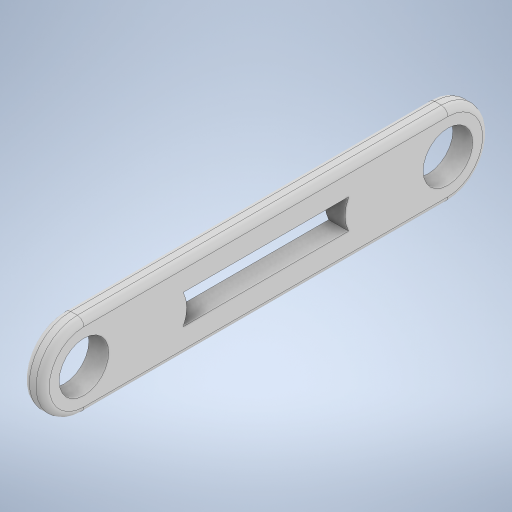
# Autodesk Inventor part: FemurHornSide
Saved by Autodesk Inventor 2024 (Build 280153000, 153)
## iProperties
Created: 2026-01-07
Part Number: FemurHornSide
Material: Generic
Document SubType Name: Modeling
Designer: Liam
Density: 1 g/cm^3
Appearance: Default
Mass: 26.103 g
Surface Area: 91.6684 cm^2
Volume: 26.103 cm^3
Author: Liam
Autodesk Inventor part; units mm, degrees
ref_plane "YZ Plane" through (0, 0, 0) normal (1, 0, 0) x (0, 1, 0)
ref_plane "XZ Plane" through (0, 0, 0) normal (0, 1, 0) x (-1, 0, 0)
ref_plane "XY Plane" through (0, 0, 0) normal (0, 0, 1) x (1, 0, 0)
sketch "Sketch1" plane through (0, 0, 0) normal (1, 0, 0) x (0, 1, 0)
  line L0 (12.5, 55) -> (-12.5, 55)
  line L1 (-12.5, 55) -> (-12.5, -55)
  line L2 (-12.5, -55) -> (12.5, -55)
  line L3 (12.5, -55) -> (12.5, 55)
  arc A0 (12.5, 55) -> (-12.5, 55) centre (0, 55) ccw
  arc A1 (-12.5, -55) -> (12.5, -55) centre (0, -55) ccw
  line L4 (4, 55) -> (-4, 55)
  circle A2 centre (0, 55) radius 7.5
  circle A3 centre (0, -55) radius 7.5
  line L5 (4.5, 25) -> (-4.5, 25)
  line L6 (-4.5, 25) -> (-4.5, -25)
  line L7 (-4.5, -25) -> (4.5, -25)
  line L8 (4.5, -25) -> (4.5, 25)
  line L9 (4.5, 25) -> (-4.5, -25) construction
  line L10 (-4.5, 25) -> (4.5, -25) construction
  arc A4 (4.5, -25) -> (-4.5, -25) centre (0, -33.9303) ccw
  arc A5 (-4.5, 25) -> (4.5, 25) centre (0, 33.9303) ccw
  point P0 (0, 0)
  point P1 (12.5, 0)
  dimension "d0" = 110
  dimension "d1" = 55
  dimension "d2" = 12.5
  dimension "d3" = 25
  dimension "d27" = 12.5
  dimension "d28" = 15
  dimension "d29" = 15
  dimension "d31" = 55
  dimension "d40" = 50
  dimension "d42" = 8
  dimension "d43" = 10
  dimension "d44" = 10
  constraints: 22 end point, 8 point on circle, 6 centre point, 6 midpoint, 4 parallel, 3 horizontal, 2 coincident, 2 perpendicular, 1 point on line
  measures "d0" distance between parallel lines of L2 L0
  measures "d1" distance from line of L2 point (0, 0)
  measures "d2" distance from line of L1 point (0, 0)
  measures "d3" distance of L1.end L2.end
  measures "d27" distance from line of L1 A0.centre
  measures "d28" diameter of A2
  measures "d29" diameter of A3
  measures "d31" distance of point (0, 0) A2.centre
  measures "d40" distance of L7.end L5.start
  measures "d42" distance between parallel lines of L1 L6
  measures "d43" radius of A5
  measures "d44" radius of A4
extrude "Extrusion1" add sketch "Sketch1" along normal blind 6 contours L3 L2 A3 L1 L0 A2 | L0 A2 A0 | A1 L2 A3 | A5 L5 | L7 A4
fillet "Fillet3" radius 2 8 edges at (6, 0, 67.5) (6, -12.5, 0) (6, 0, -67.5) (6, 12.5, 0) (0, 0, 67.5) (0, -12.5, 0) (0, 0, -67.5) (0, 12.5, 0)
equation "\"d0\" = FEMUR_X"
equation "\"d1\" = 0.5 * FEMUR_X"
equation "\"d2\" = 0.5 * FEMUR_WIDTH"
equation "\"d3\" = FEMUR_WIDTH"
equation "\"d28\" = PIVOT_DIAMETER"
equation "\"d29\" = PIVOT_DIAMETER"
equation "\"d31\" = 0.5 * FEMUR_X"
equation "\"d17\" = FEMUR_HEIGHT"
equation "\"d25\" = PART_FILLET"
equation "\"FEMUR_X\" = 110"
equation "\"FEMUR_WIDTH\" = 25"
equation "\"PIVOT_DIAMETER\" = 15"
equation "\"FEMUR_HEIGHT\" = 6"
equation "\"PART_FILLET\" = 2"
body "Solid1"
